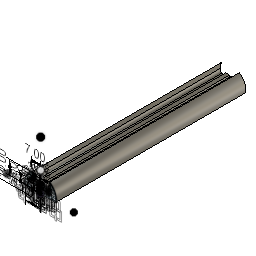
project (Autodesk Fusion 360 design; units mm, degrees)
Autodesk Fusion 360 part; units mm, degrees
sketch "Sketch1" plane through (0, 0, 0) normal (0, 1, 0) x (1, 0, 0)
  line L0 (-12.25, 0) -> (0, 0)
  line L1 (0, 0) -> (0, -15.7252) construction
  arc A0 (-12.25, 0) -> (-7, -11) centre (0, -0.9062) ccw
  arc A1 (-8.2142, -6.2319) -> (-7, -11) centre (26.2265, 0) ccw
  arc A2 (-3.925, -3.5) -> (-6.6248, -3.9119) centre (0, -38.2792) ccw
  line L2 (-3.925, -3.5) -> (-3.75, -5.5)
  line L3 (-3.75, -5.5) -> (-0.75, -5.5)
  arc A3 (-6.6248, -3.9119) -> (-8.2142, -6.2319) centre (-6.2462, -5.8758) ccw
  line L4 (-2.25, -5.5) -> (-2.25, 0) construction
  line L5 (-0.575, -3.5) -> (-0.75, -5.5)
  arc A4 (0, -3.4953) -> (-0.575, -3.5) centre (0, -38.4953) ccw
  arc A5 (8.2142, -6.2319) -> (6.6248, -3.9119) centre (6.2462, -5.8758) ccw
  arc A6 (7, -11) -> (8.2142, -6.2319) centre (-26.2265, 0) ccw
  arc A7 (7, -11) -> (12.25, 0) centre (0, -0.9062) ccw
  line L6 (12.25, 0) -> (0, 0)
  arc A8 (6.6248, -3.9119) -> (3.925, -3.5) centre (0, -38.2792) ccw
  line L7 (3.925, -3.5) -> (3.75, -5.5)
  line L8 (3.75, -5.5) -> (0.75, -5.5)
  line L9 (0.575, -3.5) -> (0.75, -5.5)
  arc A9 (0.575, -3.5) -> (0, -3.4953) centre (0, -38.4953) ccw
  dimension "d1" = 12.25
  dimension "d3" = 11
  dimension "d4" = 7
  dimension "d6" = 2
  dimension "d7" = 95
  dimension "d8" = 3
  dimension "d9" = 0.75
  dimension "d10" = 35
  dimension "d11" = 5.5
  dimension "d12" = 2
  constraint horizontal L0
  constraint coincident L0.end L1.start
  constraint vertical L1
  constraint coincident L1 A0.centre
  constraint horizontal L3
  constraint coincident A2.end A3.start
  constraint tangent A1 A3
  constraint tangent A2 A3
  constraint equal A1 A2
  constraint midpoint L3 L4.start
  constraint coincident L0 L4.end
  constraint vertical L4
  constraint symmetric A2.start L4 L5.start
  constraint symmetric L2.end L4 L3.end
  constraint coincident L1 A2.centre
  constraint coincident L1 A4.start
  constraint coincident L1 A4.centre
  constraint equal A2 A4
  constraint coincident L0 A1.centre
  constraint symmetric L0.start L1 A7.end
  constraint symmetric L0.end L1 L6.end
  constraint symmetric L1 A0.end A6.start
  constraint symmetric L1 A0 A7
  constraint symmetric L1 A2.end A5.end
  constraint symmetric L1 A1 A6
  constraint symmetric L1 A2.start A8.end
  constraint symmetric L1 A2 A8
  constraint symmetric L1 L2.end L7.end
  constraint symmetric L1 L3.end L8.end
  constraint symmetric L1 A1.start A5.start
  constraint symmetric L1 A3 A5
  constraint symmetric L1 L5.start L9.start
  constraint symmetric L1 A4.start A9.end
  constraint symmetric L1 A4 A9
  measures "d1" distance of L0.start L0.end
  measures "d3" distance of L0 A0.end
  measures "d4" distance of L1 A0.end
  measures "d6" vertical distance of A2.start L2.end
  measures "d7" angle of L2 L3
  measures "d8" distance of L2.end L3.end
  measures "d9" distance of L1 L3.end
  measures "d10" radius of A2
  measures "d11" distance of L0 L3
  measures "d12" radius of A3
extrude "Extrude1" add sketch "Sketch1" along normal blind 150
equation "d1 = ( 24.5 / 2 ) * 1 mm"
equation "d4 = ( 14 / 2 ) * 1 mm"
equation "d7 = 90 deg + 5 deg"
equation "d9 = ( 1.5 / 2 ) * 1 mm"
